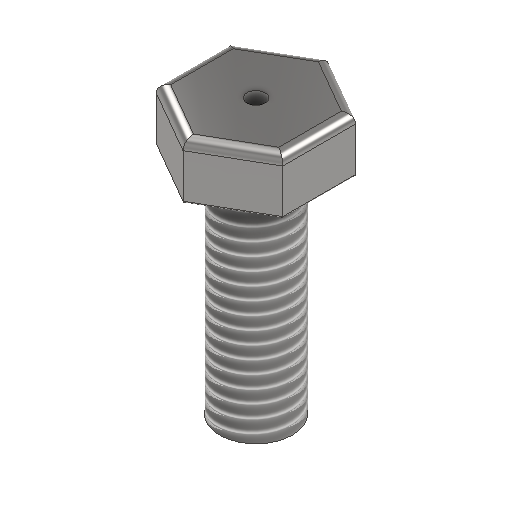
# Autodesk Inventor part: M4×12-VentedHexBolt
Saved by Autodesk Inventor 2026.2 (Build 302298000, 298)
## iProperties
Created: 2026-06-19
Part Number: M4×12-VentedHexBolt
Material: ステンレス鋼
Document SubType Name: Modeling
Designer: zetsu
Density: 8 g/cm^3
Appearance: 半つや出し
Author: zetsu
Autodesk Inventor part; units mm, degrees
ref_plane "YZ Plane" through (0, 0, 0) normal (1, 0, 0) x (0, 1, 0)
ref_plane "XZ Plane" through (0, 0, 0) normal (0, 1, 0) x (-1, 0, 0)
ref_plane "XY Plane" through (0, 0, 0) normal (0, 0, 1) x (1, 0, 0)
sketch "スケッチ1" plane through (0, 0, 0) normal (0, 1, 0) x (-1, 0, 0)
  circle A0 centre (0, 0) radius 4 construction
  line L0 (0, 0) -> (0, -4.9846) construction
  line L1 (0, 0) -> (4.0815, -2.3565) construction
  line L2 (3.4641, -2) -> (0, -4)
  line L3 (3.4641, 2) -> (3.4641, -2)
  line L4 (0, 4) -> (3.4641, 2)
  line L5 (-3.4641, 2) -> (0, 4)
  line L6 (-3.4641, -2) -> (-3.4641, 2)
  line L7 (0, -4) -> (-3.4641, -2)
  dimension "d0" = 8
  dimension "d1" = 60
  dimension "d4" = 360
  constraints: 16 end point, 2 point on circle, 2 point on line, 1 centre point, 1 coincident, 1 vertical, 19 other
  measures "d0" diameter of A0
  measures "d1" angle of L0 L1
extrude "押し出し1" add sketch "スケッチ1" along normal blind 3
fillet "フィレット1" radius 0.5 6 edges at (1.7321, 3, 3) (-1.7321, 3, 3) (-3.4641, 3, 0) (-1.7321, 3, -3) (1.7321, 3, -3) (3.4641, 3, 0)
fillet "フィレット2" radius 0.1 6 edges at (1.7321, 0, 3) (-1.7321, 0, 3) (-3.4641, 0, 0) (-1.7321, 0, -3) (1.7321, 0, -3) (3.4641, 0, 0)
sketch "スケッチ2" plane through (0, 0, 0) normal (0, -1, 0) x (1, 0, 0)
  circle A0 centre (0, 0) radius 2
  dimension "d10" = 4
  constraints: 1 centre point, 1 coincident
  measures "d10" diameter of A0
extrude "押し出し2" add sketch "スケッチ2" along normal blind 12
thread "ねじ1" size "M4x0.7" class "6g" standard "ANSI Metric M Profile" full length
sketch "スケッチ3" plane through (0, 3, 0) normal (0, 1, 0) x (1, 0, 0)
  circle A0 centre (0, 0) radius 0.5
  dimension "d15" = 1
  constraints: 1 centre point, 1 coincident
  measures "d15" diameter of A0
extrude "押し出し3" cut sketch "スケッチ3" against normal through all
